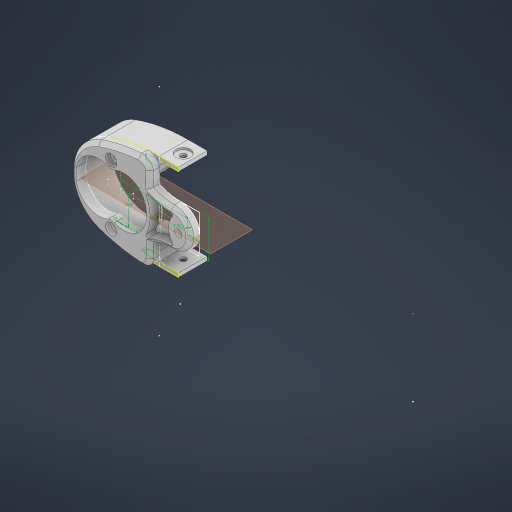
# Autodesk Inventor part: Wheel_Bracket_2
Saved by Autodesk Inventor 2024.2 (Build 282272000, 272)
## iProperties
Created: 2024-04-12
Part Number: Wheel_Bracket_2
Material: Generic
Document SubType Name: Modeling
Designer: CJ110
Density: 1 g/cm^3
Appearance: Default
Mass: 9.48645 g
Surface Area: 69.2581 cm^2
Volume: 9.48645 cm^3
Author: CJ110
## iProperties of the stored document Drive_Wheel_Bracket_3DPrint.ipt
Created: 2024-04-13
Part Number: Drive_Wheel_Bracket_3DPrint
Material: Generic
Document SubType Name: Modeling
Designer: jerem
Density: 1 g/cm^3
Appearance: Default
Author: jerem
Autodesk Inventor part; units mm, degrees
ref_plane "YZ Plane" through (0, 0, 0) normal (1, 0, 0) x (0, 1, 0)
ref_plane "XZ Plane" through (0, 0, 0) normal (0, 1, 0) x (-1, 0, 0)
ref_plane "XY Plane" through (0, 0, 0) normal (0, 0, 1) x (1, 0, 0)
sketch "Sketch1" plane through (0, 0, 0) normal (0, 0, 1) x (1, 0, 0)
  circle A0 centre (0, 0) radius 18.5
  line L0 (-30.2, 25) -> (-20.2, 25)
  line L1 (-20.2, 25) -> (-20.2, 23)
  line L2 (-20.2, 23) -> (-30.2, 23)
  line L3 (-30.2, 23) -> (-30.2, 25)
  line L4 (-30.2, -23) -> (-20.2, -23)
  line L5 (-20.2, -23) -> (-20.2, -25)
  line L6 (-20.2, -25) -> (-30.2, -25)
  line L7 (-30.2, -25) -> (-30.2, -23)
  circle A1 centre (0, 0) radius 21.5
  arc A2 (7.233339, 20.246699) -> (-20.2, 25) centre (-20.2, -56.541429) ccw
  arc A3 (-20.2, -25) -> (7.233339, -20.246699) centre (-20.2, 56.541429) ccw
  line L8 (0, 0) -> (-21.5, 0) construction
  line L9 (-20.2, 23) -> (-20.2, -23)
  point P0 (-20.2, 0)
  point P1 (-30.2, 24)
  point P2 (-17.75, 5.214163)
  point P3 (-17.75, -5.214163)
  point P4 (-20.2, -7.362744)
  point P5 (-20.2, 7.362744)
  dimension "d0" = 37
  dimension "d2" = 50
  dimension "d3" = 2
  dimension "d4" = 43
  dimension "d52" = 20.2
  dimension "d53" = 10
  constraints: 20 end point, 7 point on circle, 4 centre point, 4 parallel, 4 tangent, 3 horizontal, 3 perpendicular, 2 coincident, 2 equal length, 2 midpoint, 1 point on line
  measures "d0" diameter of A0
  measures "d2" distance between parallel lines of L6 L0
  measures "d3" distance between parallel lines of L4 L6
  measures "d4" diameter of A1
  measures "d52" distance from line of point (0, 0) L9
  measures "d53" distance between parallel lines of L9 L3
extrude "Extrusion1" add sketch "Sketch1" along normal blind 15 contours L0 L1 L2 L3 | A2 A1 L9 L1 | A1 L9 | A1 A3 L5 L9 | L5 L6 L7 L4 picked at (-19.633333, 0)
ref_plane "Work Plane1" through (-30.2, 0, 0) normal (0, 1, 0) x (1, 0, 0)
sketch "Sketch2" plane through (0, 0, 0) normal (0, 0, -1) x (-1, 0, 0)
  line L0 (0, 18.5) -> (0, -18.5) construction
  line L1 (30.2, 25) -> (30.2, 23)
  line L2 (20.2, 25) -> (30.2, 25)
  arc A0 (20.2, 25) -> (-7.233339, 20.246699) centre (20.2, -56.541429) ccw
  arc A1 (-7.233339, 20.246699) -> (-7.233339, -20.246699) centre (0, 0) ccw
  arc A2 (-7.233339, -20.246699) -> (20.2, -25) centre (20.2, 56.541429) ccw
  line L3 (30.2, -25) -> (20.2, -25)
  line L4 (30.2, -23) -> (30.2, -25)
  line L5 (20.2, -23) -> (30.2, -23)
  line L6 (20.2, 23) -> (20.2, -23)
  circle A3 centre (0, 0) radius 18.5
  line L7 (30.2, 23) -> (20.2, 23)
  circle A4 centre (0, -15.6) radius 1.27
  circle A5 centre (0, -15.6) radius 4
  arc A6 (1.651471, -11.956836) -> (18.215385, -3.232609) centre (6.545057, -1.161524) ccw
  circle A7 centre (0, 0) radius 18.5
  circle A8 centre (19.2, -3.407345) radius 1
  arc A9 (-18.215385, -3.232609) -> (-1.651471, -11.956836) centre (-6.545057, -1.161524) ccw
  circle A10 centre (0, 0) radius 21.5
  circle A11 centre (0, 0) radius 18.5
  line L8 (19.032866, -10) -> (41.2, -10)
  line L9 (41.2, -10) -> (41.2, 10)
  line L10 (41.2, 10) -> (19.032866, 10)
  circle A12 centre (35.2, 0) radius 1.905
  arc A13 (31.2, -10) -> (41.2, 0) centre (31.2, 0) ccw
  arc A14 (41.2, 0) -> (31.2, 10) centre (31.2, 0) ccw
  arc A15 (13.95364, 16.356831) -> (31.2, 10) centre (31.2, 36.573478) ccw
  arc A16 (20.2, -20) -> (23.2, -23) centre (23.2, -20) ccw
  line L11 (20.2, -23) -> (30.2, -23)
  arc A17 (21.319089, -2.783241) -> (20.2, -20) centre (153.196154, -20) ccw
  line L12 (20.2, 23) -> (20.2, -23)
  arc A18 (31.2, -10) -> (13.95364, -16.356831) centre (31.2, -36.573478) ccw
  arc A19 (23.2, 23) -> (20.2, 20) centre (23.2, 20) ccw
  arc A20 (20.2, 20) -> (21.319089, 2.783241) centre (153.196154, 20) ccw
  line L13 (20.2, 23) -> (20.2, -23)
  line L14 (20.2, 23) -> (20.2, 25)
  line L15 (20.2, -23) -> (20.2, -25)
  arc A21 (20.2, 20) -> (14.008921, 24.76463) centre (14.452694, 18.936655) ccw
  arc A22 (20.2, 25) -> (-7.233339, 20.246699) centre (20.2, -56.541429) ccw
  arc A23 (15.04701, -24.837016) -> (20.2, -20) centre (15.353296, -20) ccw
  arc A24 (-7.233339, -20.246699) -> (20.2, -25) centre (20.2, 56.541429) ccw
  line L16 (35.2, 0) -> (0, 0) construction
  circle A25 centre (0, 15.6) radius 1.27
  circle A26 centre (0, 15.6) radius 4
  arc A27 (18.215385, 3.232609) -> (1.651471, 11.956836) centre (6.545057, 1.161524) ccw
  arc A28 (-1.651471, 11.956836) -> (-18.215385, 3.232609) centre (-6.545057, 1.161524) ccw
  point P0 (17.75, -5.214163)
  point P1 (17.75, 5.214163)
  point P2 (-7.233339, 20.246699)
  point P3 (-7.233339, -20.246699)
  point P4 (-18.215385, -3.232609)
  point P5 (18.5, 0)
  point P6 (17.75, -5.214163)
  point P7 (-7.233339, 20.246699)
  point P8 (20.2, -7.362744)
  point P9 (-7.233339, -20.246699)
  point P10 (20.2, -3.407345)
  point P11 (17.75, -5.214163)
  point P12 (20.2, -10)
  point P13 (19.983889, -21.431136)
  point P14 (20.2, 12.38361)
  point P15 (-18.215385, 3.232609)
  point P16 (18.215385, 3.232609)
  dimension "d11" = 2
  dimension "d8" = 2.54
  dimension "d9" = 15.6
  dimension "d10" = 8
  dimension "d12" = 35.2
  dimension "d13" = 3.81
  dimension "d14" = 20
  dimension "d15" = 6
  dimension "d23" = 3
  dimension "d24" = 3
  constraints: 44 point on circle, 21 centre point, 21 tangent, 14 end point, 8 symmetric about line, 6 point on line, 4 coincident, 3 equal radius, 3 midpoint, 3 vertical, 2 horizontal, 2 horizontal alignment, 2 perpendicular, 1 collinear, 13 other
  measures "d8" diameter of A4
  measures "d9" distance of point (0, 0) A4.centre
  measures "d10" diameter of A5
  measures "d12" distance of point (0, 0) L16.start
  measures "d13" diameter of A12
  measures "d14" distance of L8.end L9.end
  measures "d15" distance of L16.start A13.end
  measures "d23" distance from line of L5 A16.start
  measures "d24" distance from line of L7 A19.end
extrude "Extrusion2" add sketch "Sketch2" along normal blind 5 contours A21 L6 A15 A10 A0 | A3 A5 A6 | A8 | A10 L6 A1 | A15 A20 L10 L6 | L6 L10 A10 A15 | A15 L10 A20 | A10 A18 L6 A23 A2 | L10 A20 A10 L6 | L6 A10 L10 | A14 A13 L8 A17 A10 A20 L10 | A10 L8 L6 A18 | A10 L6 | L6 A18 A17 | A10 L6 L8 | L6 L8 A17 A18 | A18 A17 L8 | A10 A17 L8 L6 | A5 A3 | A3 A5 | A27 A26 A3 | A3 A9 A5 | A26 A3 | A3 A26 | A26 A28 A3
sketch "Sketch3" plane through (0, 0, -5) normal (0, 0, -1) x (-1, 0, 0)
  circle A0 centre (0, -15.6) radius 2.95
  arc A1 (-7.233339, 20.246699) -> (-7.233339, -20.246699) centre (0, 0) ccw
  arc A2 (-7.233339, -20.246699) -> (15.04701, -24.837016) centre (20.2, 56.541429) ccw
  arc A3 (20.424078, -12.282961) -> (20.2, -20) centre (153.196154, -20) ccw
  arc A4 (31.2, -10) -> (20.424078, -12.282961) centre (31.2, -36.573478) ccw
  arc A5 (20.2, 12.38361) -> (31.2, 10) centre (31.2, 36.573478) ccw
  arc A6 (31.2, -10) -> (31.2, 10) centre (31.2, 0) ccw
  arc A7 (15.04701, -24.837016) -> (20.2, -20) centre (15.353296, -20) ccw
  line L0 (20.2, 12.38361) -> (20.2, 20)
  arc A8 (20.2, 20) -> (14.008921, 24.76463) centre (14.452694, 18.936655) ccw
  arc A9 (14.008921, 24.76463) -> (-7.233339, 20.246699) centre (20.2, -56.541429) ccw
  dimension "d20" = 5.9
  constraints: 1 centre point
  measures "d20" diameter of A0
extrude "Extrusion4" cut sketch "Sketch3" against normal blind 2.5 contours A0
mirror "Mirror2" about plane through (-30.2, 0, 0) normal (0, 1, 0) of "Extrusion4"
sketch "Sketch4" plane through (0, 0, -5) normal (0, 0, -1) x (-1, 0, 0)
  circle A0 centre (19.368732, 9) radius 1
  circle A1 centre (19.368732, -9) radius 1
  arc A2 (18.461855, -8.578605) -> (18.461855, 8.578605) centre (0, 0) ccw
  circle A3 centre (31.2, 6.568476) radius 1
  circle A4 centre (31.2, -6.568476) radius 1
  arc A5 (32.002141, 5.971342) -> (32.002141, -5.971342) centre (40.023555, 0) ccw
  arc A6 (19.779694, 9.911652) -> (31.181881, 7.568312) centre (30.700388, 34.137428) ccw
  arc A7 (31.181881, -7.568312) -> (19.779694, -9.911652) centre (30.700388, -34.137428) ccw
  line L0 (-56.439231, 0) -> (188.135385, 0)
  circle A8 centre (35.2, 0) radius 1.905
  arc A9 (18.215385, -3.232609) -> (18.215385, 3.232609) centre (0, 0) ccw
  circle A10 centre (0, 15.6) radius 2.95
  circle A11 centre (0, -15.6) radius 2.95
  arc A12 (-7.233339, 20.246699) -> (-7.233339, -20.246699) centre (0, 0) ccw
  arc A13 (-7.233339, -20.246699) -> (15.04701, -24.837016) centre (20.2, 56.541429) ccw
  arc A14 (20.424078, -12.282961) -> (20.2, -20) centre (153.196154, -20) ccw
  arc A15 (31.2, -10) -> (20.424078, -12.282961) centre (31.2, -36.573478) ccw
  arc A16 (31.2, -10) -> (31.2, 10) centre (31.2, 0) ccw
  arc A17 (20.2, 12.38361) -> (31.2, 10) centre (31.2, 36.573478) ccw
  circle A18 centre (35.2, 0) radius 1.905
  arc A19 (15.04701, -24.837016) -> (20.2, -20) centre (15.353296, -20) ccw
  arc A20 (20.2, 12.38361) -> (31.2, 10) centre (31.2, 36.573478) ccw
  line L1 (17.475209, 6.071825) -> (21.262255, 11.928175) construction
  line L2 (0, 0) -> (12.933126, 20) construction
  line L3 (19.779694, 9.911652) -> (20.779054, 12.128568) construction
  line L4 (31.181881, 7.568312) -> (31.2, 10) construction
  arc A21 (18.215385, -3.232609) -> (18.215385, 3.232609) centre (0, 0) ccw
  arc A22 (1.651471, -11.956836) -> (18.215385, -3.232609) centre (6.545057, -1.161524) ccw
  arc A23 (1.651471, -11.956836) -> (-1.651471, -11.956836) centre (0, -15.6) ccw
  arc A24 (-18.215385, -3.232609) -> (-1.651471, -11.956836) centre (-6.545057, -1.161524) ccw
  arc A25 (-18.215385, 3.232609) -> (-18.215385, -3.232609) centre (0, 0) ccw
  line L5 (20.2, 12.38361) -> (20.2, 20)
  arc A26 (20.2, 20) -> (14.008921, 24.76463) centre (14.452694, 18.936655) ccw
  arc A27 (14.008921, 24.76463) -> (-7.233339, 20.246699) centre (20.2, -56.541429) ccw
  arc A28 (-1.651471, 11.956836) -> (-18.215385, 3.232609) centre (-6.545057, 1.161524) ccw
  arc A29 (-1.651471, 11.956836) -> (1.651471, 11.956836) centre (0, 15.6) ccw
  arc A30 (18.215385, 3.232609) -> (1.651471, 11.956836) centre (6.545057, 1.161524) ccw
  point P0 (18.428622, 13.270224)
  point P1 (13.95364, 16.356831)
  point P2 (0.588886, 18.490625)
  dimension "d25" = 2
  dimension "d26" = 4
  dimension "d28" = 10
  dimension "d30" = 18
  constraints: 18 point on circle, 8 centre point, 8 end point, 8 tangent, 5 equal radius, 2 point on line, 2 vertical alignment, 1 coincident, 1 concentric, 1 equal length, 1 line through centre, 1 midpoint, 1 parallel
  measures "d25" diameter of A3
  measures "d26" horizontal distance of A4.centre A8.centre
  measures "d28" radius of A5
  measures "d30" distance of A1.centre A0.centre
extrude "Extrusion5" cut sketch "Sketch4" against normal up to surface (5 mm away) contours A0 | A0 A6 A3 A5 L0 A2 | A3 | L0 A5 A4 A7 A1 A2 | A1 | A4
sketch "Sketch5" plane through (-30.2, 25, 15) normal (0, 1, 0) x (1, 0, 0)
  circle A0 centre (5, 7.5) radius 1.59
  line L0 (10, 15) -> (0, 15) projected
  line L1 (0, 15) -> (0, 0) projected
  line L2 (10, 0) -> (0, 0) projected
  line L3 (10, 15) -> (10, 0) projected
  line L4 (0, 7.5) -> (10, 7.5) construction
  point P0 (30.2, 15)
  dimension "d36" = 3.18
  dimension "d37" = 5
  constraints: 3 midpoint, 2 end point, 1 centre point
  measures "d36" diameter of A0
  measures "d37" distance from line of L1 A0.centre
extrude "Extrusion7" cut sketch "Sketch5" against normal through all contours A0
sketch "Sketch6" plane through (-30.2, 25, 0) normal (0, 1, 0) x (1, 0, 0)
  circle A0 centre (5, -7.5) radius 1.59 projected
  line L0 (10, 0) -> (0, 0) projected
  line L1 (0, 0) -> (0, -15) projected
  line L2 (10, -15) -> (0, -15) projected
  line L3 (10, 0) -> (10, -15) projected
  circle A1 centre (5, -7.5) radius 3.75
  point P0 (30.2, 0)
  dimension "d40" = 7.5
  constraints: 1 centre point, 1 coincident
  measures "d40" diameter of A1
extrude "Extrusion8" cut sketch "Sketch6" against normal blind 1 contours A1
mirror "Mirror4" about plane through (-30.2, 0, 0) normal (0, 1, 0) of "Extrusion8"
chamfer "Chamfer1" distance 2 angle 45 10 edges at (-3.746, -23.3226, -5) (-18.6704, -23.5338, -5) (-20.256, -16.1399, -5) (21.5, 0, -5) (-3.2367, 23.216, -5) (-18.0174, 23.5686, -5) (-25.6925, -10.577, -5) (-41.2, 0, -5) (-25.5724, 10.6027, -5) (-20.2, 16.1918, -5)
sketch "Sketch9" plane through (0, 0, 15) normal (0, 0, 1) x (1, 0, 0)
  line L0 (0, 0) -> (0, 16)
  line L1 (0, 16) -> (-22, 16)
  line L2 (-22, 16) -> (-22, 0)
  line L3 (-22, 0) -> (-22, -16)
  line L4 (-22, -16) -> (0, -16)
  line L5 (0, -16) -> (0, 0)
  line L6 (-30.2, 23) -> (-20.2, 23) projected
  point P0 (-28.2, 23)
  dimension "d62" = 7
  dimension "d63" = 22
  constraints: 12 end point, 4 perpendicular, 2 collinear, 2 vertical
  measures "d62" distance between parallel lines of L6 L1
  measures "d63" distance from line of L0.start L2
extrude "Extrusion11" cut sketch "Sketch9" against normal up to surface (15 mm away)
fillet "Fillet3" radius 2 4 edges at (-20.2, 16, 7.5) (-20.2, -16, 7.5) (-9.2871, 16, 7.5) (-9.2871, -16, 7.5)
chamfer "Chamfer4" distance 1 angle 45 10 edges at (-14.0054, 16, 15) (-9.3168, 16.0619, 15) (9.4461, -15.9066, 15) (9.4461, 15.9066, 15) (-9.3168, -16.0619, 15) (-14.0054, -16, 15) (-19.6142, -16.5858, 15) (-20.2, -20.5, 15) (-19.6142, 16.5858, 15) (-20.2, 20.5, 15)
body "Solid1"
